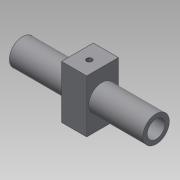
# Autodesk Inventor part: Колонка
Saved by Autodesk Inventor 2014 SP1 (Build 180222100, 222)
## iProperties
Created: 2021-12-02
Part Number: Колонка
Material: Типовые
Document SubType Name: Modeling
Designer: Украинцев
Mass: 218.675 g
Surface Area: 570.721 cm^2
Volume: 218.675 cm^3
Density: 1 g/cm^3
Appearance: По умолчанию
Author: Украинцев
Autodesk Inventor part; units mm, degrees
note: some values were not read from the file. Chosen so that the rebuilt part matches the saved one: direction of "Отверстие2"; direction of "Отверстие3"; direction of "Отверстие4".
ref_plane "YZ Plane" through (0, 0, 0) normal (1, 0, 0) x (0, 1, 0)
ref_plane "XZ Plane" through (0, 0, 0) normal (0, 1, 0) x (-1, 0, 0)
ref_plane "XY Plane" through (0, 0, 0) normal (0, 0, 1) x (1, 0, 0)
sketch "Эскиз1" plane through (0, 0, 0) normal (0, 0, 1) x (1, 0, 0)
  line L0 (-19, 24) -> (19, 24)
  line L1 (19, 24) -> (19, -24)
  line L2 (19, -24) -> (-19, -24)
  line L3 (-19, -24) -> (-19, 24)
  line L4 (-19, 24) -> (19, -24) construction
  line L5 (19, 24) -> (-19, -24) construction
  line L6 (-101, 19) -> (101, 19)
  line L7 (101, 19) -> (101, -1)
  line L8 (101, -1) -> (-101, -1)
  line L9 (-101, -1) -> (-101, 19)
  point P0 (0, 0)
  point P1 (0, 0)
  point P2 (0, -1)
  point P3 (0, 0)
  dimension "d1" = 38
  dimension "d2" = 48
  dimension "d3" = 202
  dimension "d4" = 40
  dimension "d75" = 25
  constraints: 20 end point, 4 parallel, 3 midpoint, 2 horizontal, 2 perpendicular, 1 coincident, 1 vertical alignment
  measures "d1" distance of L0.start L0.end
  measures "d2" distance of L0.end L1.end
  measures "d3" distance of L6.start L6.end
  measures "d4" diameter of L6 L8
  measures "d75" distance between parallel lines of L0 L8
extrude "Выдавливание1" add sketch "Эскиз1" along normal mid plane 80 contours L0 L1 L6 L3 | L6 L1 L8 L3 | L8 L1 L2 L3
revolve "Вращение1" add sketch "Эскиз1" angle 360 about axis through (101, -1, 0) along (-1, 0, 0) contours L6 L1 L8 L3 | L3 L8 L9 L6 | L6 L7 L8 L1
hole "Отверстие1" at (-101, -1, 0) direction (1, 0, 0) diameter 27 end through all
hole "Отверстие2" at (0, -1, -40) direction (0, 0, 1) diameter 24 end up to surface
hole "Отверстие3" at (0, -1, 40) direction (0, 0, -1) diameter 8.376 end up to surface thread size "M10x1.5" class "6H" standard "ISO Metric profile"
hole "Отверстие4" at (0, 24, 0) direction (0, -1, 0) diameter 13.835 end up to surface thread size "M16x2" class "6H" standard "ISO Metric profile"
sketch "Эскиз2" plane through (0, 0, -40) normal (0, 0, -1) x (-1, 0, 0)
  circle A0 centre (0, -1) radius 12 projected
  point P0 (12, 15)
  point P1 (-12, -17)
  point P2 (-12, 15)
  dimension "d71" = 12
  dimension "d73" = 16
  dimension "d76" = 32
  dimension "d77" = 12
  constraints: 1 horizontal alignment, 1 vertical alignment
  measures "d71" horizontal distance of A0.centre point (-12, -17)
  measures "d73" vertical distance of point (-12, -17) A0.centre
  measures "d76" distance of point (-12, 15) point (-12, -17)
  measures "d77" horizontal distance of point (12, 15) A0.centre
hole "Отверстие5" at (-12, 15, -40) at (12, -17, -40) direction (0, 0, 1) diameter 4.917 depth 14 tip angle 118 thread size "M6x1" class "6H" standard "ISO Metric profile"
hole "Отверстие6" at (12, 15, -40) direction (0, 0, 1) diameter 8 depth 22 tip angle 118
chamfer "Фаска1" distance 1 angle 45 2 edges at (-12, 12.5415, -40) (12, -19.4585, -40)
chamfer "Фаска2" distance 1.6 angle 45 1 edges at (12, 11, -40)
